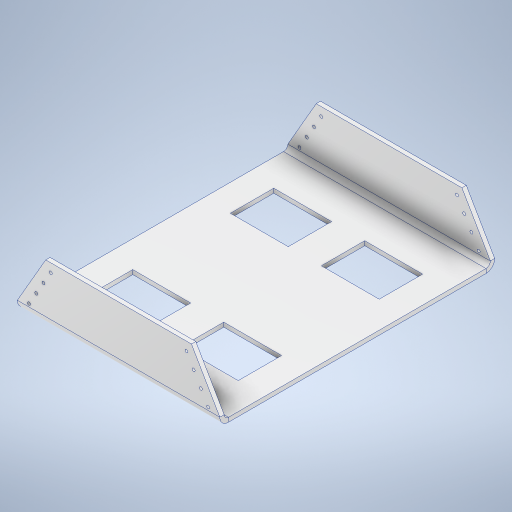
# Autodesk Inventor part: floor
Saved by Autodesk Inventor 2023 (Build 270158000, 158)
## iProperties
Created: 2022-05-09
Part Number: floor
Material: Aluminum 6061
Document SubType Name: Sheet Metal
Designer: Dan
Density: 2.7 g/cm^3
Sheet Metal Rule: Default_mm
Appearance: Aluminum - Flat
Mass: 328.217 g
Surface Area: 835.62 cm^2
Volume: 121.562 cm^3
Author: Dan
Autodesk Inventor part; units mm, degrees
ref_plane "YZ Plane" through (0, 0, 0) normal (1, 0, 0) x (0, 1, 0)
ref_plane "XZ Plane" through (0, 0, 0) normal (0, 1, 0) x (-1, 0, 0)
ref_plane "XY Plane" through (0, 0, 0) normal (0, 0, 1) x (1, 0, 0)
sketch "Sketch1" plane through (0, 0, 0) normal (0, 1, 0) x (-1, 0, 0)
  line L0 (0, 0) -> (70, 0)
  line L1 (70, 0) -> (70, -92)
  line L2 (70, -92) -> (0, -92)
  line L3 (0, -92) -> (0, 0)
  dimension "d0" = 92
  dimension "d1" = 70
  measures "d0" distance of L0.end L1.end
  measures "d1" distance of L1.end L2.end
extrude "Plate1" add sketch "Sketch1" along normal blind 3
sketch "Sketch2" plane through (0, 3, 0) normal (0, 0, 1) x (1, 0, 0)
  line L0 (-70, 0) -> (0, 0)
  line L1 (0, 0) -> (0, 37)
  line L2 (0, 37) -> (-70, 37)
  line L3 (-70, 37) -> (-70, 0)
  constraints: 6 end point, 1 horizontal, 1 perpendicular, 1 vertical
edge flange "Flange1" height 40 angle 90 thickness 3 bend radius 3 thickness toward (0, 0, 1) relief straight relief width 3 relief depth 1.5 edges at (-35, 3, 0) wall of the first edge with corners at (-70, 3, 0) (0, 3, 0) (0, 40, 0) (-70, 40, 0)
bend "Bend1"
corner "Corner1"
sketch "Sketch4" plane through (5, 0, 3) normal (0, 0, 1) x (1, 0, 0)
  circle A0 centre (-13.094, 8.0192) radius 1
  line L0 (-2.546, -10.2505) -> (-29.0222, 35.6077) construction
  circle A1 centre (-18.094, 16.6795) radius 1
  circle A2 centre (-23.094, 25.3397) radius 1
  circle A3 centre (-28.094, 34) radius 1
  line L1 (-5, 0) -> (-75, 0) projected
  line L2 (-5, 6) -> (-5, 3) projected
  line L3 (-5, 40) -> (-5, 6) projected
  line L4 (-5, 6) -> (-5, 40)
  line L5 (-5, 40) -> (-24.6299, 40)
  line L6 (-75, 40) -> (-5, 40) projected
  line L7 (-5, 0) -> (-5, 6) projected
  line L8 (-5, 6) -> (-24.6299, 40)
  point P0 (0, 34.7059)
  point P1 (-5, 3)
  dimension "d39" = 10
  dimension "d26" = 2
  dimension "d36" = 10
  dimension "d63" = 6
  dimension "d64" = 6
  dimension "d65" = 30
  constraints: 8 end point, 4 centre point, 2 point on line, 1 parallel, 1 vertical, 8 other
  measures "d26" diameter of A0
  measures "d36" distance of A0.centre A1.centre
  measures "d63" distance between parallel lines of L8 L0
  measures "d64" distance from line of L6 A3.centre
  measures "d65" angle to the sketch y axis of L8
extrude "Cut1" cut sketch "Sketch4" against normal up to next
sketch "Sketch5" plane through (0, 3, 0) normal (0, 1, 0) x (1, 0, 0)
  line L0 (-58.5515, 58.272) -> (-18.5515, 58.272)
  line L1 (-18.5515, 58.272) -> (-18.5515, 28.272)
  line L2 (-18.5515, 28.272) -> (-58.5515, 28.272)
  line L3 (-58.5515, 28.272) -> (-58.5515, 58.272)
  line L4 (28.7792, 47.5) -> (-70, 47.5) construction
  line L5 (-70, 3) -> (-70, 92) projected
  point P0 (0, 0)
  dimension "d45" = 30
  dimension "d46" = 40
  constraints: 10 end point, 2 horizontal, 2 parallel, 1 midpoint, 1 perpendicular
  measures "d45" distance of L2.end L0.start
  measures "d46" distance of L1.end L2.end
extrude "Cut2" cut sketch "Sketch5" against normal blind 3
mirror "Mirror1" about plane through (-70, 0, 0) normal (-1, 0, 0)
mirror "Mirror2" about plane through (-70, 0, -92) normal (0, 0, -1)
equation "\"d24\" = Thickness"
equation "\"d47\" = Thickness"
equation "\"d2\" = Thickness"
equation "\"d3\" = BendReliefWidth"
equation "\"d4\" = BendReliefDepth"
equation "\"d5\" = MinimumRemnant"
equation "\"d6\" = TransitionRadius"
equation "\"d9\" = BendRadius"
equation "\"d10\" = CornerReliefSize"
equation "\"d11\" = GapSize"
equation "\"d12\" = JacobiRadiusSize"
equation "\"GapSize\" = Thickness"
equation "\"BendRadius\" = Thickness"
equation "\"MinimumRemnant\" = 2 * Thickness"
equation "\"BendReliefDepth\" = 0.5 * Thickness"
equation "\"BendReliefWidth\" = Thickness"
equation "\"CornerReliefSize\" = 4 * Thickness"
equation "\"JacobiRadiusSize\" = BendRadius"
equation "\"TransitionRadius\" = BendRadius"
equation "\"Thickness\" = 3"
body "Solid1"
